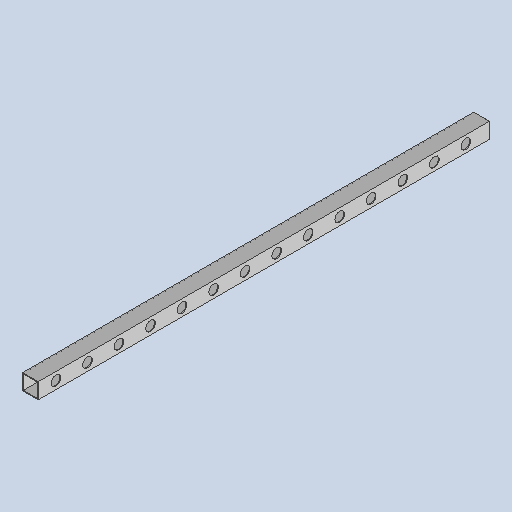
# Autodesk Inventor part: KND-1661 DrSysB way tube 1 01
Saved by Autodesk Inventor 2026.2 (Build 302298000, 298)
## iProperties
Created: 2025-06-24
Part Number: KND-1661 DrSysB way tube 1 01
Material: Stainless Steel
Document SubType Name: Modeling
Designer: admin
Mass: 1762.25 g
Surface Area: 2283.33 cm^2
Volume: 220.281 cm^3
Density: 8 g/cm^3
Sheet Metal Rule: AISI304 2mm Die16
Sheet Metal Width: 0.000 mm
Sheet Metal Length: 0.000 mm
Sheet Metal Area: 0.000 mm^2
Appearance: Default
Author: user
Autodesk Inventor part; units mm, degrees
ref_plane "YZ Plane" through (0, 0, 0) normal (1, 0, 0) x (0, 1, 0)
ref_plane "XZ Plane" through (0, 0, 0) normal (0, 1, 0) x (-1, 0, 0)
ref_plane "XY Plane" through (0, 0, 0) normal (0, 0, 1) x (1, 0, 0)
sketch "Sketch9" plane through (0, 0, 0) normal (0, 1, 0) x (-1, 0, 0)
  line L0 (20, 20) -> (-20, 20)
  line L1 (-20, 20) -> (-20, -20)
  line L2 (-20, -20) -> (20, -20)
  line L3 (20, -20) -> (20, 20)
  line L4 (20, 20) -> (-20, -20) construction
  line L5 (-20, 20) -> (20, -20) construction
  line L6 (-18, 18) -> (18, 18)
  line L7 (18, 18) -> (18, -18)
  line L8 (18, -18) -> (-18, -18)
  line L9 (-18, -18) -> (-18, 18)
  point P0 (0, 0)
  dimension "d172" = 40
  dimension "d173" = 40
  dimension "d174" = 2
  constraints: 20 end point, 4 parallel, 2 midpoint, 2 perpendicular, 1 horizontal, 3 other
  measures "d172" distance of L2.end L1.end
  measures "d173" distance of L0.end L1.end
  measures "d174" distance between parallel lines of L0 L6
extrude "Extrusion3" add sketch "Sketch9" against normal blind 1150
sketch "Sketch10" plane through (0, 0, 0) normal (1, 0, 0) x (0, 1, 0)
  line L0 (0, 20) -> (0, -20) construction
  line L1 (0, 20) -> (-1150, 20) construction
  line L2 (-1150, -20) -> (-1150, 20) construction
  line L3 (0, -20) -> (-1150, -20) construction
  circle A0 centre (-60, 0) radius 12.5
  point P0 (0, 0)
  point P1 (0, 0)
  dimension "d191" = 25
  dimension "d192" = 60
  constraints: 2 end point, 1 centre point, 1 coincident, 1 horizontal alignment, 1 midpoint
  measures "d191" diameter of A0
  measures "d192" distance of point (-60, 0) point (0, 0)
extrude "Extrusion4" cut sketch "Sketch10" along normal through all
pattern_linear "Rectangular Pattern4" count 14 spacing 80.3846 along (0, -1, 0) of "Extrusion4"
derived "KND-1401 DrSysB DIMentions 01.ipt"
body "Solid4"
